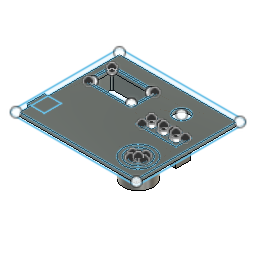
top_cover_velocitron_v1 (Autodesk Fusion 360 design; units mm, degrees)
part number: 2025-06-28-20-38-23-636
Autodesk Fusion 360 part; units mm, degrees
sketch "top_cover" plane through (0, 0, 0) normal (0, 0, 1) x (1, 0, 0)
  line L0 (-28.755, 21.4097) -> (33.245, 21.4097)
  line L1 (33.245, 21.4097) -> (33.245, -31.5903)
  line L2 (33.245, -31.5903) -> (-28.755, -31.5903)
  line L3 (-28.755, -31.5903) -> (-28.755, 21.4097)
  line L4 (34.245, -34.5903) -> (-29.755, -34.5903)
  line L5 (-31.755, -32.5903) -> (-31.755, 22.4097)
  line L6 (-29.755, 24.4097) -> (34.245, 24.4097)
  line L7 (36.245, 22.4097) -> (36.245, -32.5903)
  arc A0 (-29.755, 24.4097) -> (-31.755, 22.4097) centre (-29.755, 22.4097) ccw
  arc A1 (-31.755, -32.5903) -> (-29.755, -34.5903) centre (-29.755, -32.5903) ccw
  arc A2 (34.245, -34.5903) -> (36.245, -32.5903) centre (34.245, -32.5903) ccw
  arc A3 (36.245, 22.4097) -> (34.245, 24.4097) centre (34.245, 22.4097) ccw
  line L8 (-23.755, 13.4097) -> (-2.955, 13.4097)
  line L9 (-1.955, 12.4097) -> (-1.955, 1.9097)
  line L10 (-2.955, 0.9097) -> (-23.755, 0.9097)
  line L11 (-24.755, 1.9097) -> (-24.755, 12.4097)
  arc A4 (-23.755, 13.4097) -> (-24.755, 12.4097) centre (-23.755, 12.4097) ccw
  arc A5 (-24.755, 1.9097) -> (-23.755, 0.9097) centre (-23.755, 1.9097) ccw
  arc A6 (-2.955, 0.9097) -> (-1.955, 1.9097) centre (-2.955, 1.9097) ccw
  arc A7 (-1.955, 12.4097) -> (-2.955, 13.4097) centre (-2.955, 12.4097) ccw
  circle A8 centre (23.245, -20.5903) radius 6
  circle A9 centre (23.245, -20.5903) radius 8
  line L12 (9.245, -2.5903) -> (9.245, -1.5903)
  line L13 (14.245, -1.5903) -> (14.245, -2.5903)
  line L14 (12.245, -4.5903) -> (11.245, -4.5903)
  line L15 (11.245, 0.4097) -> (12.245, 0.4097)
  line L16 (15.745, -2.5903) -> (15.745, -1.5903)
  line L17 (20.745, -1.5903) -> (20.745, -2.5903)
  line L18 (18.745, -4.5903) -> (17.745, -4.5903)
  line L19 (17.745, 0.4097) -> (18.745, 0.4097)
  line L20 (24.245, 0.4097) -> (25.245, 0.4097)
  line L21 (27.245, -1.5903) -> (27.245, -2.5903)
  line L22 (25.245, -4.5903) -> (24.245, -4.5903)
  line L23 (22.245, -2.5903) -> (22.245, -1.5903)
  line L24 (7.745, 1.9097) -> (28.745, 1.9097)
  line L25 (28.745, 1.9097) -> (28.745, -6.0903)
  line L26 (28.745, -6.0903) -> (7.745, -6.0903)
  line L27 (7.745, -6.0903) -> (7.745, 1.9097)
  arc A10 (11.245, 0.4097) -> (9.245, -1.5903) centre (11.245, -1.5903) ccw
  arc A11 (9.245, -2.5903) -> (11.245, -4.5903) centre (11.245, -2.5903) ccw
  arc A12 (12.245, -4.5903) -> (14.245, -2.5903) centre (12.245, -2.5903) ccw
  arc A13 (14.245, -1.5903) -> (12.245, 0.4097) centre (12.245, -1.5903) ccw
  arc A14 (17.745, 0.4097) -> (15.745, -1.5903) centre (17.745, -1.5903) ccw
  arc A15 (15.745, -2.5903) -> (17.745, -4.5903) centre (17.745, -2.5903) ccw
  arc A16 (18.745, -4.5903) -> (20.745, -2.5903) centre (18.745, -2.5903) ccw
  arc A17 (20.745, -1.5903) -> (18.745, 0.4097) centre (18.745, -1.5903) ccw
  arc A18 (24.245, 0.4097) -> (22.245, -1.5903) centre (24.245, -1.5903) ccw
  arc A19 (22.245, -2.5903) -> (24.245, -4.5903) centre (24.245, -2.5903) ccw
  arc A20 (25.245, -4.5903) -> (27.245, -2.5903) centre (25.245, -2.5903) ccw
  arc A21 (25.1873, -17.2262) -> (19.3605, -20.5903) centre (23.245, -20.5903) ccw
  arc A22 (24.3028, -18.7582) -> (25.1873, -17.2262) centre (24.745, -17.9922) ccw
  arc A23 (24.3028, -18.7582) -> (21.1295, -20.5903) centre (23.245, -20.5903) ccw
  arc A24 (19.3605, -20.5903) -> (21.1295, -20.5903) centre (20.245, -20.5903) ccw
  arc A25 (24.745, -17.9922) -> (20.245, -20.5903) centre (23.245, -20.5903) ccw construction
  arc A26 (21.2877, -23.9804) -> (27.1596, -20.5903) centre (23.245, -20.5903) ccw
  arc A27 (22.2023, -22.3964) -> (21.2877, -23.9804) centre (21.745, -23.1884) ccw
  arc A28 (22.2023, -22.3964) -> (25.3304, -20.5903) centre (23.245, -20.5903) ccw
  arc A29 (27.1596, -20.5903) -> (25.3304, -20.5903) centre (26.245, -20.5903) ccw
  arc A30 (21.745, -23.1884) -> (26.245, -20.5903) centre (23.245, -20.5903) ccw construction
  line L28 (23.245, -20.5903) -> (21.745, -23.1884) construction
  line L29 (23.245, -20.5903) -> (26.245, -20.5903) construction
  line L30 (-30.755, -16.5903) -> (-21.755, -16.5903)
  line L31 (-21.755, -16.5903) -> (-21.755, -25.5903)
  line L32 (-21.755, -25.5903) -> (-30.755, -25.5903)
  line L33 (-30.755, -25.5903) -> (-30.755, -16.5903)
  circle A31 centre (15.245, 10.4097) radius 4
  arc A32 (27.245, -1.5903) -> (25.245, 0.4097) centre (25.245, -1.5903) ccw
  arc A33 (-0.955, 12.4097) -> (-2.955, 14.4097) centre (-2.955, 12.4097) ccw
  line L34 (-23.755, 14.4097) -> (-2.955, 14.4097)
  arc A34 (-23.755, 14.4097) -> (-25.755, 12.4097) centre (-23.755, 12.4097) ccw
  line L35 (-25.755, 1.9097) -> (-25.755, 12.4097)
  arc A35 (-25.755, 1.9097) -> (-23.755, -0.0903) centre (-23.755, 1.9097) ccw
  line L36 (-2.955, -0.0903) -> (-23.755, -0.0903)
  arc A36 (-2.955, -0.0903) -> (-0.955, 1.9097) centre (-2.955, 1.9097) ccw
  line L37 (-0.955, 12.4097) -> (-0.955, 1.9097)
  point P0 (-24.755, 13.4097)
  point P1 (-1.955, 13.4097)
  point P2 (-24.755, 0.9097)
  point P3 (9.245, 0.4097)
  point P4 (9.245, -4.5903)
  point P5 (14.245, 0.4097)
  point P6 (15.745, 0.4097)
  point P7 (20.745, 0.4097)
  point P8 (22.245, 0.4097)
  point P9 (27.245, 0.4097)
  dimension "d1" = 62
  dimension "d2" = 53
  dimension "d4" = 2
  dimension "d5" = 2
  dimension "d6" = 2
  dimension "d7" = 2
  dimension "d8" = 22.8
  dimension "d9" = 12.5
  dimension "d10" = 1
  dimension "d11" = 1
  dimension "d12" = 1
  dimension "d13" = 1
  dimension "d14" = 4
  dimension "d15" = 8
  dimension "d16" = 12
  dimension "d17" = 10
  dimension "d18" = 11
  dimension "d19" = 2
  dimension "d33" = 5
  dimension "d34" = 5
  dimension "d37" = 5
  dimension "d41" = 1.5
  dimension "d42" = 5
  dimension "d44" = 1.5
  dimension "d46" = 21
  dimension "d47" = 8
  dimension "d48" = 1.5
  dimension "d49" = 1.5
  dimension "d50" = 4.5
  dimension "d51" = 19.5
  dimension "d52" = 1.5
  dimension "d53" = 1.5
  dimension "d54" = 2
  dimension "d55" = 3
  dimension "d56" = 3
  dimension "d57" = 120
  dimension "d58" = 9
  dimension "d59" = 9
  dimension "d60" = 1
  dimension "d61" = 6
  dimension "d62" = 8
  dimension "d63" = 11
  dimension "d64" = 18
  dimension "d69" = 2
  dimension "d78" = -1
  dimension "d95" = 5
  dimension "d96" = 5
  constraint horizontal L0
  constraint vertical L1
  constraint horizontal L2
  constraint vertical L3
  constraint tangent L5 A0
  constraint tangent L6 A0
  constraint tangent L4 A1
  constraint tangent L5 A1
  constraint tangent L4 A2
  constraint tangent L7 A2
  constraint tangent L6 A3
  constraint tangent L7 A3
  constraint horizontal L8
  constraint vertical L9
  constraint horizontal L10
  constraint vertical L11
  constraint coincident P0 L8
  constraint coincident P0 L11
  constraint tangent L8 A4
  constraint tangent L11 A4
  constraint coincident P2 L10
  constraint coincident P2 L11
  constraint tangent L10 A5
  constraint tangent L11 A5
  constraint tangent L9 A6
  constraint tangent L10 A6
  constraint coincident P1 L8
  constraint coincident P1 L9
  constraint tangent L8 A7
  constraint tangent L9 A7
  constraint horizontal L15
  constraint vertical L13
  constraint horizontal L14
  constraint vertical L12
  constraint horizontal L19
  constraint vertical L17
  constraint horizontal L18
  constraint vertical L16
  constraint horizontal L20
  constraint vertical L21
  constraint horizontal L22
  constraint vertical L23
  constraint horizontal L24
  constraint vertical L25
  constraint horizontal L26
  constraint vertical L27
  constraint coincident P3 L12
  constraint coincident P3 L15
  constraint tangent L12 A10
  constraint tangent L15 A10
  constraint coincident P4 L12
  constraint coincident P4 L14
  constraint tangent L12 A11
  constraint tangent L14 A11
  constraint equal A10 A11
  constraint tangent L13 A12
  constraint tangent L14 A12
  constraint equal A10 A12
  constraint coincident P5 L13
  constraint coincident P5 L15
  constraint tangent L13 A13
  constraint tangent L15 A13
  constraint equal A10 A13
  constraint coincident P6 L16
  constraint coincident P6 L19
  constraint tangent L16 A14
  constraint tangent L19 A14
  constraint equal A10 A14
  constraint tangent L16 A15
  constraint tangent L18 A15
  constraint equal A10 A15
  constraint tangent L17 A16
  constraint tangent L18 A16
  constraint equal A10 A16
  constraint coincident P7 L17
  constraint coincident P7 L19
  constraint tangent L17 A17
  constraint tangent L19 A17
  constraint equal A10 A17
  constraint coincident P8 L20
  constraint coincident P8 L23
  constraint tangent L20 A18
  constraint tangent L23 A18
  constraint equal A10 A18
  constraint tangent L22 A19
  constraint tangent L23 A19
  constraint equal A10 A19
  constraint tangent L21 A20
  constraint tangent L22 A20
  constraint equal A10 A20
  constraint tangent A21 A22
  constraint tangent A22 A23
  constraint tangent A23 A24
  constraint tangent A21 A24
  constraint coincident A8.centre A9.centre
  constraint tangent A26 A27
  constraint tangent A27 A28
  constraint tangent A28 A29
  constraint tangent A26 A29
  constraint horizontal L30
  constraint vertical L31
  constraint horizontal L32
  constraint vertical L33
  constraint coincident P9 L20
  constraint coincident P9 L21
  constraint tangent L20 A32
  constraint tangent L21 A32
  measures "d1" distance of L0.start L0.end
  measures "d2" distance of L0.start L2.end
  measures "d4" radius of A0
  measures "d5" radius of A1
  measures "d6" radius of A2
  measures "d7" radius of A3
  measures "d8" distance of P0 P1
  measures "d9" distance of P0 P2
  measures "d10" radius of A4
  measures "d11" radius of A5
  measures "d12" radius of A6
  measures "d13" radius of A7
  measures "d14" distance of L3 L11
  measures "d15" distance of L0 L8
  measures "d16" diameter of A8
  measures "d17" distance of L1 A8.centre
  measures "d18" distance of L2 A8.centre
  measures "d33" distance of P3 P5
  measures "d34" distance of P3 P4
  measures "d37" distance of P6 P7
  measures "d41" distance of L13 L16
  measures "d42" distance of P8 P9
  measures "d44" distance of L17 L23
  measures "d46" distance of L24.start L24.end
  measures "d47" distance of L24.start L26.end
  measures "d48" distance of L12 L27
  measures "d49" distance of L15 L24
  measures "d50" distance of L1 L25
  measures "d51" distance of L0 L24
  measures "d52" distance of L19 L24
  measures "d53" distance of L20 L24
  measures "d54" radius of A10
  measures "d55" radius of A25
  measures "d56" radius of A30
  measures "d57" angle of L28 L29
  measures "d58" distance of L30.start L30.end
  measures "d59" distance of L30.start L32.end
  measures "d60" distance of L5 L33
  measures "d61" distance of L2 L32
  measures "d62" diameter of A31
  measures "d63" distance of L0 A31.centre
  measures "d64" distance of L1 A31.centre
  measures "d69" radius of A32
  measures "d95" distance of L18 L19
  measures "d96" distance of L20 L22
extrude "Extrude1" add sketch "top_cover" against normal blind 20 contours L4 L5 L6 L7 A0 A1 A2 A3 makes body 1
extrude "Extrude2" add sketch "top_cover" against normal blind 2 contours L0 L1 L2 L3 L30 L31 L32 | A33 L34 A34 L35 A35 L36 A36 L37 bodies 1
extrude "Extrude3" add sketch "top_cover" against normal blind 10 contours L24 L25 L26 L27 bodies 1
extrude "Extrude4" add sketch "top_cover" against normal blind 5 contours A9 bodies 1
extrude "Extrude5" add sketch "top_cover" against normal blind 1 contours A8 bodies 1
extrude "Extrude6" add sketch "top_cover" against normal blind 1 contours L3 L30 L31 L32 | L3 L30 L32 L33 bodies 1
extrude "Extrude7" add sketch "top_cover" against normal blind 4 separate body contours A33 L34 A34 L35 A35 L36 A36 L37 makes body 2
extrude "Extrude8" add sketch "top_cover" against normal blind 20 separate body contours L4 L5 L6 L7 A0 A1 A2 A3 makes body 3
extrude "Extrude9" add sketch "top_cover" against normal blind 2 separate body contours L0 L1 L2 L3 L30 L31 L32 | L3 L30 L31 L32 | A8 | A9 | L24 L25 L26 L27 | A33 L34 A34 L35 A35 L36 A36 L37 makes body 4
extrude "Extrude10" add sketch "top_cover" against normal blind 10 separate body contours A9 makes body 5
extrude "Extrude12" add sketch "top_cover" against normal blind 2 contours L3 L30 L32 L33 bodies 4
extrude "Extrude13" add sketch "top_cover" against normal blind 10 separate body contours A33 L34 A34 L35 A35 L36 A36 L37 makes body 6
extrude "Extrude14" add sketch "top_cover" against normal blind 10 separate body contours L24 L25 L26 L27 makes body 7
hidden bodies 1 2 3
named bodies: "top_cover", "outter_wall", "face_plate", "speaker_slot", "displya_slot", "led_slot"
